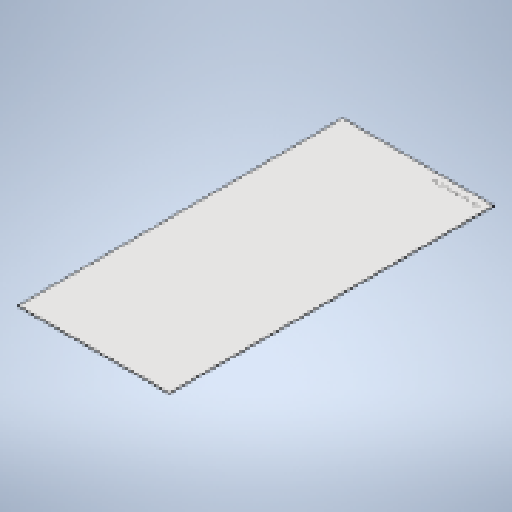
# Autodesk Inventor part: TRM 011 bottom main
Saved by Autodesk Inventor 2025.1 (Build 291241020, 241B)
## iProperties
Created: 2024-08-07
Part Number: TRM 011 bottom main
Material: AISI 304
Document SubType Name: Sheet Metal
Designer: pokla
Density: 8.02768 g/cm^3
Flat Pattern Width: 81 cm
Flat Pattern Length: 49 cm
Flat Pattern Area: 3969 cm^2
Sheet Metal Rule: AISI304 2mm Die16
Sheet Metal Width: 810.000 mm
Sheet Metal Length: 490.000 mm
Sheet Metal Area: 396900.000 mm^2
Appearance: Default
Stock Number: ТРМ 011 дно основное
Author: pokla
Autodesk Inventor part; units mm, degrees
ref_plane "YZ Plane" through (0, 0, 0) normal (1, 0, 0) x (0, 1, 0)
ref_plane "XZ Plane" through (0, 0, 0) normal (0, 1, 0) x (-1, 0, 0)
ref_plane "XY Plane" through (0, 0, 0) normal (0, 0, 1) x (1, 0, 0)
sketch "Sketch1" plane through (0, 0, 0) normal (0, 0, 1) x (1, 0, 0)
  line L0 (-245, -405) -> (245, -405)
  line L1 (245, -405) -> (245, 405)
  line L2 (245, 405) -> (-245, 405)
  line L3 (-245, 405) -> (-245, -405)
  line L4 (-245, -405) -> (245, 405) construction
  line L5 (245, -405) -> (-245, 405) construction
  point P0 (0, 0)
  dimension "d0" = 490
  dimension "d1" = 810
  measures "d0" distance of L2.end L1.end
  measures "d1" distance of L1.end L0.end
extrude "Plate1" add sketch "Sketch1" along normal blind 2
sketch "Sketch2" plane through (0, 0, 0) normal (0, 0, -1) x (-1, 0, 0)
  line L0 (-245, 405) -> (245, 405) projected
  line L1 (-245, -405) -> (-245, 405) projected
  line L2 (-225, 385) -> (-25, 385) construction
  line L3 (-25, 385) -> (-25, 365) construction
  line L4 (-25, 365) -> (-225, 365) construction
  line L5 (-225, 365) -> (-225, 385) construction
  point P0 (0, 0)
  dimension "d8" = 200
  dimension "d9" = 20
  dimension "d10" = 20
  dimension "d11" = 20
  constraints: 2 other
  measures "d8" distance of L2.start L2.end
  measures "d9" distance of L2.end L3.end
  measures "d10" distance between parallel lines of L0 L2
  measures "d11" distance between parallel lines of L1 L5
mark "Mark3"
equation "\"d2\" = Thickness"
equation "\"BendReliefWidth\" = Thickness"
equation "\"BendReliefDepth\" = 0.5 * Thickness"
equation "\"CornerReliefSize\" = 4 * Thickness"
equation "\"MinimumRemnant\" = 2 * Thickness"
equation "\"TransitionRadius\" = BendRadius"
equation "\"JacobiRadiusSize\" = BendRadius"
equation "\"GapSize\" = Thickness"
equation "\"Thickness\" = 2"
equation "\"BendRadius\" = 2.75"
body "Solid1"
